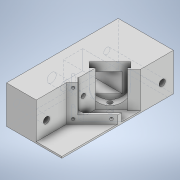
# Autodesk Inventor part: minimal micro scanner 2
Saved by Autodesk Inventor 2022 (Build 260153000, 153)
## iProperties
Created: 2023-08-23
Part Number: minimal micro scanner 2
Material: Generic
Document SubType Name: Modeling
Designer: William
Density: 1 g/cm^3
Appearance: Default
Author: William
Autodesk Inventor part; units mm, degrees
ref_plane "YZ Plane" through (0, 0, 0) normal (1, 0, 0) x (0, 1, 0)
ref_plane "XZ Plane" through (0, 0, 0) normal (0, 1, 0) x (-1, 0, 0)
ref_plane "XY Plane" through (0, 0, 0) normal (0, 0, 1) x (1, 0, 0)
sketch "Sketch1" plane through (0, 0, 0) normal (0, 1, 0) x (-1, 0, 0)
  line L0 (24.505382, -20) -> (6.505382, -20) construction
  line L1 (6.505382, -20) -> (6.505382, -29.5) construction
  line L2 (6.505382, -29.5) -> (24.505382, -29.5) construction
  line L3 (0, -36.005382) -> (10.505382, -25.5)
  line L4 (11.313708, -13.494618) -> (0, -24.808326)
  line L5 (8.505382, -18) -> (0, -26.505382)
  line L6 (8.505382, -18) -> (10.505382, -18)
  line L7 (0, 0) -> (24.505382, 0)
  line L8 (24.505382, 0) -> (24.505382, -49.5)
  line L9 (24.505382, -49.5) -> (0, -49.5)
  line L10 (0, -49.5) -> (0, 0)
  line L11 (6.505382, -20) -> (5.656854, -19.151472) construction
  line L12 (10.505382, -18) -> (10.505382, -25.5)
  line L13 (11.313708, -13.494618) -> (11.313708, 0)
  line L14 (2.727208, -33.278175) -> (5.06066, -35.611627)
  line L15 (5.06066, -35.611627) -> (14.253048, -26.419239)
  line L16 (14.253048, -26.419239) -> (11.919596, -24.085786)
  line L17 (7.323402, -28.681981) -> (9.656854, -31.015433)
  line L18 (10.505382, -25.5) -> (11.919596, -24.085786)
  line L19 (3.434315, -32.571068) -> (2.868629, -32.005382)
  line L20 (2.868629, -32.005382) -> (0, -34.874012)
  circle A0 centre (8.490128, -29.848707) radius 1
  line L21 (24.505382, -20) -> (10.505382, -20)
  line L22 (24.505382, -22) -> (18.505382, -22)
  line L23 (18.505382, -22) -> (18.505382, -20.6)
  line L24 (18.505382, -20.6) -> (15.505382, -20.6)
  line L25 (15.505382, -20.6) -> (15.505382, -21)
  line L26 (15.505382, -21) -> (10.505382, -21)
  dimension "d0" = 45
  dimension "d1" = 45
  dimension "d2" = 1.2
  dimension "d3" = 2
  dimension "d4" = 14
  dimension "d5" = 8
  dimension "d6" = 8
  dimension "d9" = 20
  dimension "d10" = 20
  dimension "d11" = 9.5
  dimension "d12" = 3.3
  dimension "d13" = 13
  dimension "d14" = 2
  dimension "d46" = 2
  dimension "d49" = 0.8
  dimension "d50" = 1
  dimension "d51" = 2
  dimension "d52" = 1
  dimension "d53" = 0.6
  dimension "d54" = 5
  dimension "d55" = 6
  dimension "d56" = 2
  constraints: 54 end point, 17 point on line, 15 perpendicular, 4 horizontal, 4 parallel, 3 midpoint, 2 vertical, 1 centre point
  measures "d0" angle of L0 L5
  measures "d1" angle of L1 L3
  measures "d2" distance between parallel lines of L5 L4
  measures "d3" distance between parallel lines of L0 L6
  measures "d4" distance between parallel lines of L8 L12
  measures "d5" distance from line of L4.start L11
  measures "d6" distance from line of L4.end L11
  measures "d9" distance between parallel lines of L9 L2
  measures "d10" distance between parallel lines of L7 L0
  measures "d11" distance between parallel lines of L0 L2
  measures "d12" distance of L15.end L16.end
  measures "d13" distance of L14.end L15.end
  measures "d14" distance of L5.start L6.end
  measures "d46" distance of L3.end L16.end
  measures "d49" distance of L19.start L19.end
  measures "d50" distance between parallel lines of L14 L19
  measures "d51" diameter of A0
  measures "d52" distance between parallel lines of L0 L26
  measures "d53" distance between parallel lines of L0 L24
  measures "d54" distance of L25.end L26.end
  measures "d55" distance of L22.start L22.end
  measures "d56" distance between parallel lines of L0 L22
extrude "Extrusion1" add sketch "Sketch1" along normal blind 8 and the other way blind 10 contours L10 L20 L19 L3 | L3 L14 L15 L16 L18 L12 L26 L25 L24 L23 L22 L8 L9 L10 | L3 L17 A0 L15 L14 | L10 L5 L6 L12 L3 L19 L20 | L10 L4 L13 L7 L8 L21 L12 L6 L5 | L3 L18 L16 L15 L17 A0 | L22 L23 L24 L25 L26 L12 L21 L8 | L10 L7 L13 L4
extrude "Extrusion2" cut sketch "Sketch1" along normal blind 13 and the other way blind 8 contours L10 L5 L6 L12 L3 L19 L20 | L10 L7 L13 L4
revolve "Revolution2" cut sketch "Sketch1" angle 360 about axis through (-24.505382, 0, -20) along (1, 0, 0) contours L22 L23 L24 L25 L26 L12 L21 L8
extrude "Extrusion3" cut sketch "Sketch1" along normal blind 13 contours L3 L17 A0 L15 L14 | L3 L18 L16 L15 L17 A0 | A0 L17 | L17 A0
revolve "Revolution1" cut sketch "Sketch1" angle 360 about axis through (-7.323402, 0, -28.681981) along (-0.7071068, 0, -0.7071068) picked at (8.589296, -30.166947) contours L3 L17 A0 L15 L14 | L17 A0
sketch "Sketch2" plane through (-24.505382, -10, 0) normal (-1, 0, 0) x (0, 0, 1)
  line L0 (-33.75, 5.75) -> (-25.25, 5.75)
  line L1 (-25.25, 5.75) -> (-25.25, 14.25)
  line L2 (-25.25, 14.25) -> (-33.75, 14.25)
  line L3 (-33.75, 14.25) -> (-33.75, 5.75)
  circle A0 centre (-20, 10) radius 1
  circle A1 centre (-20, 10) radius 2
  circle A2 centre (-44.5, 8) radius 1.397
  circle A3 centre (-4.5, 8) radius 1.397
  point P0 (0, 10)
  point P1 (-20, 10)
  point P2 (-20, 10)
  point P3 (-20, 10)
  point P4 (-29.5, 10)
  point P5 (-29.5, 10)
  point P6 (-29.5, 10)
  point P7 (-33.75, 10)
  point P8 (-29.5, 14.25)
  dimension "d24" = 8.5
  dimension "d25" = 15.5
  dimension "d26" = 2
  dimension "d27" = 2.794
  dimension "d28" = 15
  dimension "d29" = 4
  dimension "d30" = 2
  constraints: 8 end point, 4 centre point, 2 coincident, 2 horizontal alignment, 2 midpoint, 2 parallel, 2 perpendicular, 1 equal radius, 1 horizontal, 1 vertical alignment
  measures "d24" distance of L0.end L1.end
  measures "d25" horizontal distance of A3.centre point (-20, 10)
  measures "d26" vertical distance of A3.centre point (-20, 10)
  measures "d27" diameter of A3
  measures "d28" horizontal distance of A2.centre point (-29.5, 10)
  measures "d29" diameter of A1
  measures "d30" diameter of A0
extrude "Extrusion4" cut sketch "Sketch2" against normal up to next contours L3 L2 L1 L0 | A2 | A3
sketch "Sketch3" plane through (-11.313708, -8, -13.494618) normal (0.7071068, 0, 0.7071068) x (0.7071068, 0, -0.7071068)
  line L0 (2, 2) -> (14, 2) construction
  line L1 (14, 2) -> (14, 14) construction
  line L2 (14, 14) -> (2, 14) construction
  line L3 (2, 14) -> (2, 2) construction
  line L4 (3.5, 3.5) -> (19.455942, 3.5)
  line L5 (19.455942, 3.5) -> (19.455942, 23.765103)
  line L6 (19.455942, 23.765103) -> (3.5, 23.765103)
  line L7 (3.5, 23.765103) -> (3.5, 3.5)
  circle A0 centre (2, 2) radius 0.6
  circle A1 centre (2, 14) radius 0.6
  circle A2 centre (14, 2) radius 0.6
  point P0 (-1.542136, 8)
  point P1 (8, 8)
  point P2 (8, 8)
  point P3 (8, 8)
  point P4 (14, 8)
  point P5 (8, 14)
  dimension "d35" = 4.5
  dimension "d36" = 4.5
  dimension "d37" = 12
  dimension "d38" = 1.2
  constraints: 16 end point, 4 parallel, 3 centre point, 3 coincident, 3 perpendicular, 2 equal radius, 2 horizontal, 2 midpoint, 1 horizontal alignment, 1 vertical alignment
  measures "d35" distance from line of L7 point (8, 8)
  measures "d36" distance from line of L4 point (8, 8)
  measures "d37" distance of L0.end L1.end
  measures "d38" diameter of A0
extrude "Extrusion6" cut sketch "Sketch3" against normal blind 2.7 contours L7 L6 L5 L4
extrude "Extrusion7" cut sketch "Sketch3" against normal blind 7 contours A0 | A1 | A2
chamfer "Chamfer1" distance 1.27 angle 45 4 edges at (-12.2527, -10, -49.5) (0, -10, -24.75) (-24.5054, -10, -24.75) (-12.2527, -10, 0)
body "Solid1"
